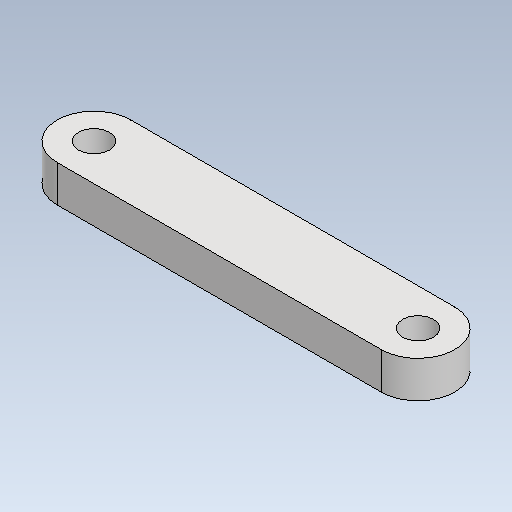
# Autodesk Inventor part: upper-tipper-link
Saved by Autodesk Inventor 2025 (Build 290162000, 162)
## iProperties
Created: 2025-08-20
Part Number: upper-tipper-link
Material: Generic
Document SubType Name: Modeling
Designer: HP
Density: 1 g/cm^3
Appearance: Default
Author: HP
Autodesk Inventor part; units mm, degrees
ref_plane "YZ Plane" through (0, 0, 0) normal (1, 0, 0) x (0, 1, 0)
ref_plane "XZ Plane" through (0, 0, 0) normal (0, 1, 0) x (-1, 0, 0)
ref_plane "XY Plane" through (0, 0, 0) normal (0, 0, 1) x (1, 0, 0)
sketch "Sketch1" plane through (0, 0, 0) normal (0, 1, 0) x (-1, 0, 0)
  line L0 (22, 0) -> (-22, 0) construction
  line L1 (22, 5) -> (-22, 5)
  line L2 (-22, -5) -> (22, -5)
  arc A0 (22, -5) -> (22, 5) centre (22, 0) ccw
  arc A1 (-22, 5) -> (-22, -5) centre (-22, 0) ccw
  circle A2 centre (22, 0) radius 2.1
  circle A3 centre (-22, 0) radius 2.1
  point P0 (0, 0)
  point P1 (0, 0)
  dimension "d0" = 10
  dimension "d1" = 4.2
  dimension "d2" = 4.2
  dimension "d3" = 44
  constraints: 8 end point, 4 centre point, 4 point on circle, 4 tangent, 3 coincident, 1 horizontal, 1 midpoint, 1 parallel
  measures "d0" diameter of A1
  measures "d1" diameter of A2
  measures "d2" diameter of A3
  measures "d3" distance of L0.start L0.end
extrude "Extrusion1" add sketch "Sketch1" along normal blind 5
body "Solid1"
